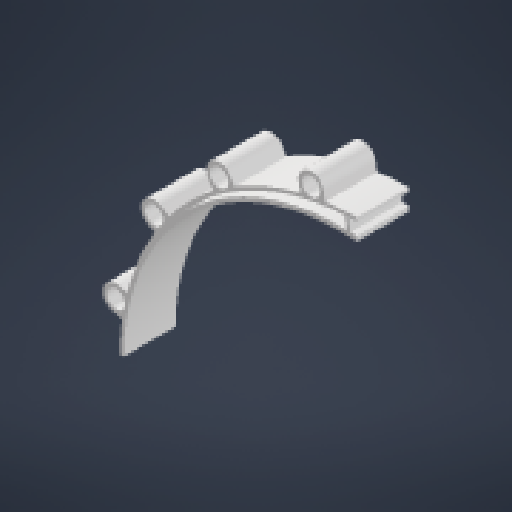
# Autodesk Inventor part: HalfFilterwall
Saved by Autodesk Inventor 2026 (Build 300175050, 175E)
## iProperties
Created: 2026-05-05
Part Number: HalfFilterwall
Material: Generic
Document SubType Name: Modeling
Designer: sniel
Density: 1 g/cm^3
Appearance: Default
Author: sniel
Autodesk Inventor part; units mm, degrees
ref_plane "YZ Plane" through (0, 0, 0) normal (1, 0, 0) x (0, 1, 0)
ref_plane "XZ Plane" through (0, 0, 0) normal (0, 1, 0) x (-1, 0, 0)
ref_plane "XY Plane" through (0, 0, 0) normal (0, 0, 1) x (1, 0, 0)
sketch "Sketch1" plane through (0, 0, 0) normal (0, 0, 1) x (1, 0, 0)
  line L0 (114.0018, -96.7355) -> (117.0413, -96.7355)
  arc A0 (117.0413, -96.7355) -> (-105.1806, -30.8316) centre (-9, -114.1273) ccw
  arc A1 (134.2355, -114.2355) -> (-105.1806, -30.8316) centre (0, -114.2355) ccw
  line L1 (134.2355, -114.2355) -> (136.2355, -114.2355)
  arc A2 (136.2355, -114.2355) -> (135.007, -95.8653) centre (0, -114.1197) ccw
  line L2 (135.007, -95.8653) -> (139.9434, -95.0589)
  arc A3 (139.9434, -95.0589) -> (137.1339, -80.3297) centre (138.7343, -87.657) ccw
  line L3 (137.1339, -80.3297) -> (132.2473, -81.397)
  arc A4 (132.2473, -81.397) -> (116.6514, -43.7451) centre (0, -114.1197) ccw
  line L4 (116.6514, -43.7451) -> (120.8614, -41.0445)
  arc A5 (120.8614, -41.0445) -> (112.4329, -28.6428) centre (116.8119, -34.7317) ccw
  line L5 (112.4329, -28.6428) -> (108.3722, -31.5631)
  arc A6 (108.3722, -31.5631) -> (82.5566, -5.7475) centre (0, -114.1197) ccw
  line L6 (82.5566, -5.7475) -> (85.4769, -1.6867)
  arc A7 (85.4769, -1.6867) -> (73.0752, 6.7417) centre (79.388, 2.6922) ccw
  line L7 (73.0752, 6.7417) -> (70.3746, 2.5317)
  arc A8 (70.3746, 2.5317) -> (32.7226, 18.1276) centre (0, -114.1197) ccw
  line L8 (32.7226, 18.1276) -> (33.7899, 23.0142)
  arc A9 (33.7899, 23.0142) -> (19.0608, 25.8237) centre (26.4627, 24.6146) ccw
  line L9 (19.0608, 25.8237) -> (18.2544, 20.8873)
  arc A10 (18.2544, 20.8873) -> (-18.2544, 20.8873) centre (0, -114.1201) ccw
  line L10 (-18.2544, 20.8873) -> (-19.0608, 25.8237)
  arc A11 (-19.0608, 25.8237) -> (-33.79, 23.0142) centre (-26.4627, 24.6146) ccw
  line L11 (-33.79, 23.0142) -> (-32.7227, 18.1276)
  arc A12 (-32.7227, 18.1276) -> (-70.3746, 2.5317) centre (0, -114.1197) ccw
  line L12 (-70.3746, 2.5317) -> (-73.0753, 6.7417)
  arc A13 (-73.0753, 6.7417) -> (-85.477, -1.6867) centre (-79.3881, 2.6922) ccw
  line L13 (-85.477, -1.6867) -> (-82.5566, -5.7475)
  arc A14 (-82.5566, -5.7475) -> (-108.3722, -31.5631) centre (0, -114.1197) ccw
  line L14 (-108.3722, -31.5631) -> (-112.433, -28.6428)
  arc A15 (-112.433, -28.6428) -> (-120.8615, -41.0445) centre (-116.8119, -34.7317) ccw
  line L15 (-120.8615, -41.0445) -> (-116.6514, -43.7451)
  arc A16 (-116.6514, -43.7451) -> (-132.2473, -81.397) centre (0, -114.1197) ccw
  line L16 (-132.2473, -81.397) -> (-137.134, -80.3297)
  arc A17 (-137.134, -80.3297) -> (-139.9435, -95.0589) centre (-138.7343, -87.657) ccw
  line L17 (-139.9435, -95.0589) -> (-135.0071, -95.8653)
  arc A18 (-135.0071, -95.8653) -> (-136.2355, -114.2355) centre (0, -114.1197) ccw
  line L18 (-136.2355, -114.2355) -> (-134.2355, -114.2355)
  arc A19 (114.0018, -96.7355) -> (-134.2355, -114.2355) centre (-9.5, -114.2355) ccw
  circle A20 centre (138.7343, -87.7729) radius 5.25
  circle A21 centre (116.8119, -34.8475) radius 5.25
  circle A22 centre (26.4627, 24.4988) radius 5.25
  circle A23 centre (79.388, 2.5764) radius 5.25
  circle A24 centre (-138.7343, -87.7729) radius 5.25
  circle A25 centre (-116.8119, -34.8475) radius 5.25
  circle A26 centre (-79.388, 2.5764) radius 5.25
  circle A27 centre (-26.4627, 24.4988) radius 5.25
  line L19 (0, 22.1158) -> (0, 10.1377)
  line L20 (-3.7531, 13) -> (-5.752, 13.0668)
  line L21 (-5.752, 13.0668) -> (-7, 19.8174)
  line L22 (-7, 19.8174) -> (-5.002, 19.9068)
  line L23 (-5.002, 19.9068) -> (-3.7531, 13)
  point P0 (0, 0)
  point P1 (0, 12.7895)
  point P2 (0, 20)
  dimension "d2" = 2
  dimension "d3" = 2
  constraints: 48 end point, 46 point on circle, 28 centre point
  measures "d2" distance of L20.start L20.end
  measures "d3" distance of L21.end L22.end
extrude "Extrusion1" add sketch "Sketch1" along normal blind 30 contours A19 L18 A18 L17 A17 L16 A16 L15 A15 L14 A14 L13 A13 L12 A12 L11 A11 L10 A10 L19 A1 A0 L20 | L20 A0 | A0 L21 L22 L23 | L22 A1
body "Solid1"
